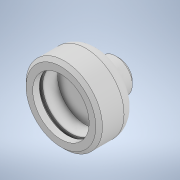
# Autodesk Inventor part: Practica 5
Saved by Autodesk Inventor 2020.2 (Build 242310000, 310)
## iProperties
Created: 2020-02-17
Part Number: Practica 5
Material: Genérico
Document SubType Name: Chapa
Designer: Luis Gallardo
Density: 1 g/cm^3
Sheet Metal Rule: Por defecto_mm
Appearance: Valor por defecto
Author: Luis Gallardo
Autodesk Inventor part; units mm, degrees
ref_plane "YZ Plane" through (0, 0, 0) normal (1, 0, 0) x (0, 1, 0)
ref_plane "XZ Plane" through (0, 0, 0) normal (0, 1, 0) x (-1, 0, 0)
ref_plane "XY Plane" through (0, 0, 0) normal (0, 0, 1) x (1, 0, 0)
sketch "Boceto1" plane through (0, 0, 0) normal (0, 1, 0) x (-1, 0, 0)
  line L0 (0, 0) -> (17, 0) construction
  line L1 (17, -15) -> (0, -15)
  line L2 (0, -15) -> (0, -35)
  line L3 (0, -35) -> (8, -35)
  line L4 (10, -33) -> (10, -23)
  line L5 (10, -23) -> (15, -23)
  line L6 (23, -15) -> (23, -2)
  line L7 (8, -35) -> (10, -33)
  arc A0 (15, -23) -> (23, -15) centre (15, -15) ccw
  line L8 (21, 0) -> (17, 0)
  line L9 (23, -2) -> (21, 0)
  line L10 (17, 0) -> (17, -4) construction
  line L11 (17, -4) -> (19, -4)
  line L12 (19, -4) -> (19, -6)
  line L13 (19, -6) -> (17, -6)
  line L14 (17, 0) -> (17, -4)
  line L15 (17, -6) -> (17, -15)
  point P0 (10, -35)
  point P1 (23, 0)
  point P2 (23, 0)
  dimension "d2" = 17
  dimension "d4" = 2
  dimension "d5" = 45
  dimension "d11" = 8
  dimension "d13" = 23
  dimension "d14" = 10
  dimension "d15" = 10
  dimension "d17" = 15
  dimension "d18" = 2
  dimension "d19" = 45
  dimension "d20" = 35
  dimension "d21" = 4
  dimension "d22" = 2
  dimension "d23" = 2
  dimension "d24" = 9
  constraints: 32 end point, 13 perpendicular, 7 point on line, 2 point on circle, 2 tangent, 1 centre point, 1 collinear, 1 horizontal, 1 vertical
  measures "d2" distance of L0.start L0.end
  measures "d4" distance of L3.end point (10, -35)
  measures "d5" angle of L3 L7
  measures "d11" radius of A0
  measures "d13" distance between parallel lines of L6 L2
  measures "d14" distance between parallel lines of L4 L2
  measures "d15" distance of L4.start L4.end
  measures "d17" distance of L0.end L1.start
  measures "d18" distance of L6.end point (23, 0)
  measures "d19" angle of L6 L9
  measures "d20" distance between parallel lines of L8 L3
  measures "d21" distance of L0.end L10.end
  measures "d22" distance of L10.end L11.end
  measures "d23" distance of L11.end L12.end
  measures "d24" distance of L13.end L1.start
revolve "Revolución1" add sketch "Boceto1" angle 360 about axis through (0, 0, -15) along (0, 0, -1)
equation "\"Radio_pliegue\" = Grosor"
equation "\"Anchura_desahogo_plegado\" = Grosor"
equation "\"Profundidad_desahogo_plegado\" = 0.5 * Grosor"
equation "\"Tamaño_destalonado\" = 4 * Grosor"
equation "\"Remanente_mínimo\" = 2 * Grosor"
equation "\"Radiodetransición\" = Radio_pliegue"
equation "\"Tamaño_de_radio_de_Jacobi\" = Radio_pliegue"
equation "\"TamañoSeparación\" = Grosor"
equation "\"Grosor\" = 0.5"
